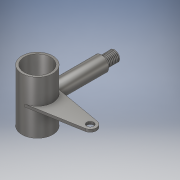
# Autodesk Inventor part: steering_kingpin_right
Saved by Autodesk Inventor 2019 (Build 230136000, 136)
## iProperties
Created: 2019-04-24
Part Number: steering_kingpin_right
Material: Steel, Mild
Document SubType Name: Modeling
Designer: callum.snowden
Density: 7.85 g/cm^3
Appearance: Semi-Polished
Author: callum.snowden
Autodesk Inventor part; units mm, degrees
sketch "Sketch1" plane through (0, 0, 0) normal (0, 1, 0) x (-1, 0, 0)
  line L0 (0, -24.5) -> (0, 24.5) construction
  line L1 (-24.5, 0) -> (24.5, 0) construction
  circle A0 centre (0, 0) radius 17.5
  circle A1 centre (0, 0) radius 15
  dimension "d0" = 35
  dimension "d1" = 30
  constraints: 2 centre point, 2 coincident
  measures "d0" diameter of A0
  measures "d1" diameter of A1
extrude "Extrusion1" add sketch "Sketch1" along normal blind 60
ref_plane "Work Plane5" through (17.5, 0, 0) normal (1, 0, 0) x (0, 1, 0)
ref_plane "Work Plane6" through (0, 30, 0) normal (0, -1, 0) x (1, 0, 0)
sketch "Sketch7" plane through (0, 30, 0) normal (0, -1, 0) x (1, 0, 0)
  circle A0 centre (0, 0) radius 15 construction
  line L0 (0, 24.5) -> (0, -24.5) construction
  line L1 (-34.4, 0) -> (83.9, 0) construction
  arc A1 (61.225, -6.892) -> (61.225, 6.892) centre (60, 0) ccw
  line L2 (3.0625, -17.2299) -> (61.225, -6.892)
  line L3 (3.0625, 17.2299) -> (61.225, 6.892)
  arc A2 (3.0625, -17.2299) -> (3.0625, 17.2299) centre (0, 0) ccw
  circle A3 centre (60, 0) radius 4
  dimension "d35" = 14
  dimension "d36" = 60
  dimension "d37" = 8
  constraints: 4 centre point, 4 end point, 4 point on circle, 4 tangent, 1 coincident, 1 point on line
  measures "d35" diameter of A1
  measures "d36" distance of A1.centre point (0, 0)
  measures "d37" diameter of A3
extrude "Extrusion5" add sketch "Sketch7" along normal mid plane 3
ref_plane "Work Plane7" through (0, 0, -17.5) normal (0, 0, 1) x (1, 0, 0)
sketch "Sketch8" plane through (0, 0, -17.5) normal (0, 0, 1) x (1, 0, 0)
  circle A0 centre (0, 25) radius 6 projected
  circle A1 centre (0, 25) radius 8.5 projected
  point P0 (0, 0)
extrude "Extrusion6" add sketch "Sketch8" against normal blind 55 contours A0 | A1
extrude "Extrusion7" add sketch "Sketch8" against normal blind 70 contours A0
extrude "Extrusion8" add sketch "Sketch8" along normal up to next contours A0 | A1
thread "Thread2" size "M12x1.75" class "6g" standard "ANSI Metric M Profile" full length
equation "\"d23\" = 55deg"
equation "\"Sketch4_Pitch\" = 1.75"
body "Solid1"
